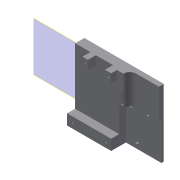
# Autodesk Inventor part: 10_Baseplate_Minispim
Saved by Autodesk Inventor 2019 (Build 230136000, 136)
## iProperties
Created: 2019-08-20
Part Number: 10_Baseplate_Minispim
Material: Generic
Document SubType Name: Modeling
Designer: diederichbenedict
Density: 1 g/cm^3
Appearance: Default
Author: diederichbenedict
Autodesk Inventor part; units mm, degrees
ref_plane "YZ Plane" through (0, 0, 0) normal (1, 0, 0) x (0, 1, 0)
ref_plane "XZ Plane" through (0, 0, 0) normal (0, 1, 0) x (-1, 0, 0)
ref_plane "XY Plane" through (0, 0, 0) normal (0, 0, 1) x (1, 0, 0)
ref_plane "Work Plane2" through (0, 0, -28.1) normal (0, 0, -1) x (-1, 0, 0)
sketch "Sketch3" plane through (0, 0, -28.1) normal (0, 0, -1) x (-1, 0, 0)
  arc A0 (-145, 50.55) -> (-153, 42.55) centre (-145, 42.55) ccw construction
  line L0 (73, 36.65) -> (73, -36.65) construction
  line L1 (75, -38.65) -> (75, 38.65) construction
  line L2 (-75, -38.65) -> (75, -38.65) construction
  line L3 (75, 38.65) -> (-75, 38.65) construction
  line L4 (-133, 53.55) -> (-3, 53.55)
  line L5 (-3, 53.55) -> (-3, -56.45)
  line L6 (-3, -56.45) -> (-133, -56.45)
  line L7 (-133, -56.45) -> (-133, 53.55)
  point P0 (0, 0)
  dimension "d0" = 130
  dimension "d1" = 110
  dimension "d2" = 3
  dimension "d3" = 20
  constraints: 8 end point, 2 parallel, 1 horizontal, 1 perpendicular
  measures "d0" distance of L5.end L6.end
  measures "d1" distance of L4.end L5.end
  measures "d2" distance from line of A0.start L4
  measures "d3" distance from line of A0.end L7
extrude "Extrusion1" add sketch "Sketch3" against normal up to surface (4 mm away)
sketch "Sketch4" plane through (3, 53.55, -28.1) normal (0, 1, 0) x (1, 0, 0)
  line L0 (140, -8.6) -> (93, -8.6) projected
  arc A0 (93, -8.6) -> (83, -18.6) centre (93, -18.6) ccw projected
  line L1 (83, -18.6) -> (83, -22.6) projected
  arc A1 (150, -18.6) -> (140, -8.6) centre (140, -18.6) ccw projected
  line L2 (93, -18.6) -> (140, -18.6) construction
  line L3 (93, -28.6) -> (140, -28.6)
  line L4 (140, -8.6) -> (93, -8.6)
  arc A2 (93, -8.6) -> (93, -28.6) centre (93, -18.6) ccw
  arc A3 (140, -28.6) -> (140, -8.6) centre (140, -18.6) ccw
  line L5 (82.5, -22.6) -> (82.5, -18.6)
  arc A4 (93, -8.1) -> (82.5, -18.6) centre (93, -18.6) ccw
  line L6 (93, -8.1) -> (140, -8.1)
  arc A5 (150.5, -18.6) -> (140, -8.1) centre (140, -18.6) ccw
  line L7 (0, -4) -> (130, -4) projected
  line L8 (130, -4) -> (130, -8.1)
  line L9 (82.5, -18.6) -> (72, -18.6)
  line L10 (72, -26.1) -> (72, -17) projected
  line L11 (72, -18.6) -> (72, -4)
  line L12 (70, -15) -> (-76, -15) construction
  line L13 (72, -15) -> (0, -15)
  line L14 (0, -4) -> (0, -15)
  point P0 (-3, -28.1)
  point P1 (116.5, -18.6)
  dimension "d6" = 0.5
  constraints: 22 end point, 8 point on circle, 5 point on line, 4 centre point, 4 tangent, 2 horizontal, 2 perpendicular, 1 concentric, 1 midpoint, 1 parallel, 1 vertical, 3 other
  measures "d6" distance between parallel lines of L0 L6
ref_plane "Work Plane3" through (88.7803, 5.45, -16.4) normal (0, -1, 0) x (1, 0, 0)
extrude "Extrusion2" add sketch "Sketch4" against normal up to surface (48.1 mm away) contours A4 L9 L10 L11 L7 L8 L6 | L11 L13 L14 L7
sketch "Sketch6" plane through (133, -56.45, -24.1) normal (0, 0, 1) x (1, 0, 0)
  circle A0 centre (-45.95, 29.8) radius 1.575 projected
  circle A1 centre (-23.8, 27.975) radius 1.575 projected
  circle A2 centre (-21.1, 55.3691) radius 0.9 projected
  circle A3 centre (-21.1, 55.3691) radius 2
  circle A4 centre (-37.8, 8.65) radius 0.9
  circle A5 centre (-48.1, 54.5) radius 0.9
  circle A6 centre (-37.8, 8.65) radius 2
  circle A7 centre (-48.1, 54.5) radius 2
  point P0 (-133, 56.45)
  dimension "d13" = 4
  dimension "d16" = 4
  dimension "d17" = 4
  constraints: 5 centre point, 3 coincident, 4 other
  measures "d13" diameter of A3
  measures "d16" diameter of A6
  measures "d17" diameter of A7
ref_plane "Work Plane4" through (106.2, -5.55, -21.8) normal (0, 0, -1) x (0, 1, 0)
extrude "Extrusion4" add sketch "Sketch6" along normal up to surface (2.3 mm away) contours A2 | A3 | A4 | A5 | A6 | A7
sketch "Sketch7" plane through (95.2, -47.8, -21.8) normal (0, 0, 1) x (1, 0, 0)
  circle A0 centre (0, 0) radius 2 projected
  point P0 (-95.2, 47.8)
ref_plane "Work Plane5" through (85.2, -49.8, -20.6) normal (0, 0, -1) x (0, 1, 0)
extrude "Extrusion5" add sketch "Sketch7" along normal up to surface (1.2 mm away)
sketch "Sketch8" plane through (133, -56.45, -24.1) normal (0, 0, 1) x (1, 0, 0)
  circle A0 centre (-37.8, 8.65) radius 2 projected
  circle A1 centre (-21.1, 55.3691) radius 2 projected
  arc A2 (-46.1, 54.5) -> (-46.1, 54.5) centre (-48.1, 54.5) ccw projected
  circle A3 centre (-37.8, 8.65) radius 2 projected
  circle A4 centre (-48.1, 54.5) radius 2 projected
  circle A5 centre (-21.1, 55.3691) radius 2 projected
  line L0 (0, 61.9) -> (-130, 61.9) projected
  line L1 (-130, 61.9) -> (-130, 0) projected
  line L2 (-130, 0) -> (0, 0) projected
  line L3 (0, 0) -> (0, 61.9) projected
  line L4 (-15.0573, 47.2459) -> (-15.0573, 52.2459) projected
  line L5 (-15.0573, 52.2459) -> (0, 52.2459) projected
  line L6 (0, 52.2459) -> (0, 47.2459) projected
  line L7 (0, 47.2459) -> (-15.0573, 47.2459) projected
  line L8 (-48.1502, 0) -> (-48.1502, 17.3563) projected
  line L9 (-43.1502, 17.3563) -> (-43.1502, 0) projected
  line L10 (-48.1502, 17.3563) -> (-43.1502, 17.3563) projected
  point P0 (-133, 56.45)
  point P1 (-2.1794, 49.7459)
  point P2 (-10.9357, 49.7459)
  point P3 (-45.6502, 2.4045)
  point P4 (-45.6502, 13.604)
hole "Hole1" at (95.2, -47.8, -24.1) at (84.9, -1.95, -24.1) at (111.9, -1.0809, -24.1) at (87.3498, -54.0455, -24.1) at (87.3498, -42.846, -24.1) at (122.0643, -6.7041, -24.1) at (130.8206, -6.7041, -24.1) direction (0, 0, -1) diameter 1.9 end through all both
sketch "Sketch9" plane through (3, -56.45, -24.1) normal (0, 0, 1) x (1, 0, 0)
  line L0 (0, 61.9) -> (72, 61.9) projected
  line L1 (72, 110) -> (72, 61.9) projected
  line L2 (0, 110) -> (72, 110) projected
  line L3 (0, 110) -> (0, 61.9) projected
  circle A0 centre (78.05, 34.75) radius 1.45 construction
  line L4 (74.2, 23.4395) -> (74.2, 36.5) construction
  line L5 (74.2, 36.5) -> (75.6, 36.5) construction
  line L6 (75.6, 36.5) -> (75.6, 25.8) construction
  arc A1 (75.6, 25.8) -> (77.3, 24.1) centre (77.3, 25.8) ccw construction
  line L7 (77.3, 24.1) -> (83.3, 24.1) construction
  line L8 (83.3, 24.1) -> (83.3, 22.45) construction
  line L9 (83.3, 22.45) -> (74.7713, 22.45) construction
  line L10 (74.7713, 22.45) -> (74.2, 23.4395) construction
  line L11 (90.2, 10.65) -> (97.8, 10.65) construction
  line L12 (97.8, 10.65) -> (97.8, 9.15) construction
  line L13 (97.8, 9.15) -> (101, 9.15) construction
  line L14 (101, 9.15) -> (101, 19.45) construction
  line L15 (101, 19.45) -> (117, 19.45) construction
  line L16 (117, 19.45) -> (117, 21.45) construction
  line L17 (117, 21.45) -> (119.1132, 21.45) construction
  line L18 (119.1132, 21.45) -> (122, 26.45) construction
  line L19 (122, 26.45) -> (122, 35.45) construction
  line L20 (122, 35.45) -> (112.7, 35.45) construction
  line L21 (112.7, 35.45) -> (112.7, 34.75) construction
  line L22 (112.7, 34.75) -> (108.7, 34.75) construction
  line L23 (108.7, 34.75) -> (108.7, 53.25) construction
  line L24 (108.7, 53.25) -> (107.7, 53.25) construction
  line L25 (107.7, 53.25) -> (107.7, 33.25) construction
  line L26 (107.7, 33.25) -> (108.7, 33.25) construction
  line L27 (108.7, 33.25) -> (108.7, 23.5) construction
  line L28 (108.7, 23.5) -> (102.2, 23.5) construction
  line L29 (102.2, 23.5) -> (102.2, 24.8) construction
  line L30 (102.2, 24.8) -> (77.3, 24.8) construction
  arc A2 (76.3, 25.8) -> (77.3, 24.8) centre (77.3, 25.8) ccw construction
  line L31 (76.3, 25.8) -> (76.3, 31.8) construction
  arc A3 (76.8, 32.3) -> (76.3, 31.8) centre (76.8, 31.8) ccw construction
  line L32 (76.8, 32.3) -> (78.05, 32.3) construction
  arc A4 (78.05, 32.3) -> (80.5, 34.75) centre (78.05, 34.75) ccw construction
  line L33 (80.5, 34.75) -> (80.5, 35.3) construction
  arc A5 (80.5, 35.3) -> (78.5, 37.3) centre (78.5, 35.3) ccw construction
  line L34 (78.5, 37.3) -> (73.4, 37.3) construction
  line L35 (73.4, 37.3) -> (73.4, 22.8251) construction
  line L36 (73.4, 22.8251) -> (74.1939, 21.45) construction
  line L37 (74.1939, 21.45) -> (82.2, 21.45) construction
  arc A6 (90.2, 13.45) -> (82.2, 21.45) centre (82.2, 13.45) ccw construction
  line L38 (90.2, 13.45) -> (90.2, 10.65) construction
  line L39 (89, 54.0921) -> (89, 60.7459) construction
  arc A7 (89, 60.7459) -> (87, 60.0519) centre (95.8767, 37.6997) ccw construction
  line L40 (87, 60.0519) -> (87, 56.0519) construction
  line L41 (87, 56.0519) -> (83.1981, 52.25) construction
  line L42 (83.1981, 52.25) -> (80.1981, 52.25) construction
  line L43 (80.1981, 52.25) -> (80.1981, 54.75) construction
  line L44 (72, 54.75) -> (80.1981, 54.75) construction
  line L45 (72, 37.3) -> (72, 54.75) construction
  line L46 (78.5, 37.3) -> (72, 37.3) construction
  arc A8 (80.5, 35.3) -> (78.5, 37.3) centre (78.5, 35.3) ccw construction
  line L47 (80.5, 49.8) -> (80.5, 35.3) construction
  line L48 (84.7079, 49.8) -> (80.5, 49.8) construction
  line L49 (84.7079, 49.8) -> (89, 54.0921) construction
  line L50 (0, 0) -> (130, 0) construction
  line L51 (0, 61.9) -> (72, 61.9) construction
  line L52 (72, 61.9) -> (72, 0) construction
  line L53 (72, 0) -> (0, 0) construction
  line L54 (0, 0) -> (0, 61.9) construction
  line L55 (0, 61.9) -> (0, 0) projected
  line L56 (0, 0) -> (72, 0)
  line L57 (72, 0) -> (72, 61.9)
  line L58 (72, 61.9) -> (0, 61.9)
  line L59 (0, 61.9) -> (0, 0)
  point P0 (-3, 56.45)
  constraints: 16 end point, 4 parallel, 2 horizontal, 2 perpendicular, 1 point on line
extrude "Extrusion6" add sketch "Sketch9" along normal up to surface (11 mm away) contours L0 L57 L56 L55
sketch "Sketch10" plane through (3, 53.55, -13.1) normal (0, 0, 1) x (1, 0, 0)
  line L0 (72, 0) -> (72, -48.1) construction
  line L1 (0, 0) -> (72, 0) construction
  line L2 (0, -110) -> (0, 0) construction
  line L3 (72, -110) -> (0, -110) construction
  line L4 (72, -48.1) -> (72, -110) construction
  line L5 (-78, -92.2) -> (72, -92.2) construction
  line L6 (72, -14.9) -> (-78, -14.9) construction
  line L7 (72, 0) -> (61.9, 0)
  line L8 (61.9, 0) -> (61.9, -14.4)
  line L9 (61.9, -14.4) -> (72, -14.4)
  line L10 (72, -14.4) -> (72, 0)
  line L11 (0, 0) -> (72, 0) projected
  line L12 (72, -110) -> (130, -110) projected
  line L13 (0, 0) -> (0, -110) projected
  line L14 (72, -110) -> (0, -110)
  line L15 (0, -110) -> (0, -92.7)
  line L16 (0, -92.7) -> (72, -92.7)
  line L17 (72, -92.7) -> (72, -110)
  line L18 (58.9, -14.9) -> (37, -14.9) projected
  line L19 (58.9, -14.9) -> (58.9, -28) projected
  line L20 (58.9, -28) -> (37, -28) projected
  line L21 (37, -14.9) -> (37, -28) projected
  line L22 (22, -14.9) -> (2, -14.9) projected
  line L23 (22, -14.9) -> (22, -28) projected
  line L24 (22, -28) -> (2, -28) projected
  line L25 (2, -14.9) -> (2, -28) projected
  line L26 (34, 0) -> (25, 0)
  line L27 (25, 0) -> (25, -14.4)
  line L28 (25, -14.4) -> (34, -14.4)
  line L29 (34, -14.4) -> (34, 0)
  point P0 (-3, -53.55)
  dimension "d29" = 0.5
  dimension "d31" = 3
  dimension "d32" = 3
  dimension "d33" = 3
  constraints: 24 end point, 6 parallel, 3 horizontal, 3 perpendicular, 2 point on line
  measures "d29" distance between parallel lines of L16 L5
  measures "d31" distance between parallel lines of L19 L8
  measures "d32" distance between parallel lines of L29 L21
  measures "d33" distance between parallel lines of L23 L27
ref_plane "Work Plane6" through (-73, -36.65, 0) normal (0, 0, 1) x (1, 0, 0)
extrude "Extrusion7" add sketch "Sketch10" along normal up to surface (13.1 mm away) contours L10 L9 L8 L7 | L11 L29 L28 L27 | L16 L17 L14 L13
sketch "Sketch11" plane through (0, 0, -28.1) normal (0, 0, -1) x (-1, 0, 0)
  line L0 (-75, 5.45) -> (-85.5, 5.45) projected
  line L1 (-85.5, 53.55) -> (-85.5, 5.45) projected
  line L2 (-75, 53.55) -> (-85.5, 53.55) projected
  line L3 (-75, 53.55) -> (-75, 39.15) projected
  line L4 (-75, 39.15) -> (-75, 5.45) projected
  line L5 (-85.5, 53.55) -> (-85.5, 5.45) projected
  line L6 (-85.5, 8.4413) -> (-82.3028, 8.4413)
  line L7 (-82.3028, 8.4413) -> (-82.3028, 27.8547)
  line L8 (-82.3028, 27.8547) -> (-85.5, 27.8547)
  line L9 (-85.5, 27.8547) -> (-85.5, 8.4413)
  point P0 (0, 0)
  constraints: 8 end point, 2 parallel, 1 horizontal, 1 perpendicular, 1 point on line
extrude "Extrusion8" cut sketch "Sketch11" against normal through all contours L1 L8 L7 L6
sketch "Sketch12" plane through (3, -39.15, 0) normal (0, 0, 1) x (1, 0, 0)
  line L0 (0, 0) -> (72, 0) projected
  line L1 (0, -17.3) -> (0, 0) projected
  line L2 (72, -17.3) -> (0, -17.3) projected
  line L3 (72, 0) -> (72, -17.3) projected
  line L4 (25, 78.3) -> (25, 92.7) projected
  line L5 (34, 92.7) -> (34, 78.3) projected
  line L6 (25, 92.7) -> (34, 92.7) projected
  line L7 (25, 78.3) -> (25, 92.7) projected
  line L8 (34, 78.3) -> (25, 78.3) projected
  line L9 (72, 92.7) -> (72, 78.3) projected
  line L10 (61.9, 92.7) -> (72, 92.7) projected
  line L11 (61.9, 78.3) -> (61.9, 92.7) projected
  line L12 (72, 78.3) -> (61.9, 78.3) projected
  circle A0 centre (8.65, -8.65) radius 8.65
  circle A1 centre (63.35, -8.65) radius 8.65
  circle A2 centre (26.8, 85.5) radius 7.2
  circle A3 centre (69.1, 85.5) radius 7.2
  point P0 (-3, 39.15)
  point P1 (29.5, 85.5)
  point P2 (66.95, 85.5)
  constraints: 12 tangent, 4 centre point
hole "Hole2" at (11.65, -47.8, 0) at (66.35, -47.8, 0) at (32.5, 46.35, 0) at (69.95, 46.35, 0) direction (0, 0, -1) diameter 2.8 end through all both
sketch "Sketch13" plane through (3, -39.15, 0) normal (0, 0, 1) x (1, 0, 0)
  line L0 (18.1086, 2.1288) -> (58.1608, 2.1288)
  line L1 (58.1608, 2.1288) -> (58.1608, -5.8817)
  line L2 (58.1608, -5.8817) -> (18.1086, -5.8817)
  line L3 (18.1086, -5.8817) -> (18.1086, 2.1288)
  point P0 (-3, 39.15)
  constraints: 8 end point, 2 parallel, 1 horizontal, 1 perpendicular
extrude "Extrusion9" cut sketch "Sketch13" against normal up to surface (13.1 mm away)
sketch "Sketch14" plane through (0, 0, -28.1) normal (0, 0, -1) x (-1, 0, 0)
  point P0 (0, 0)
body "Solid1"
